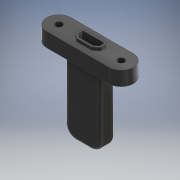
# Autodesk Inventor part: hdmi-panel-mount
Saved by Autodesk Inventor 2017 (Build 210142000, 142)
## iProperties
Created: 2020-10-05
Part Number: hdmi-panel-mount
Material: Generic
Document SubType Name: Modeling
Designer: Joe Ferner
Density: 1 g/cm^3
Appearance: Default
Author: Joe Ferner
Autodesk Inventor part; units mm, degrees
ref_plane "YZ Plane" through (0, 0, 0) normal (1, 0, 0) x (0, 1, 0)
ref_plane "XZ Plane" through (0, 0, 0) normal (0, 1, 0) x (-1, 0, 0)
ref_plane "XY Plane" through (0, 0, 0) normal (0, 0, 1) x (1, 0, 0)
sketch "Sketch1" plane through (0, 0, 0) normal (0, 0, 1) x (1, 0, 0)
  line L0 (0, 0) -> (43.8634, 0)
  line L1 (43.8634, 17.0268) -> (0, 17.0268)
  arc A0 (0, 17.0268) -> (0, 0) centre (0, 8.5134) ccw
  arc A1 (43.8634, 0) -> (43.8634, 17.0268) centre (43.8634, 8.5134) ccw
  circle A2 centre (0, 8.5134) radius 2.3193
  circle A3 centre (43.8634, 8.5134) radius 2.3193
  dimension "d0" = 43.8634
  dimension "d1" = 17.0268
  dimension "d2" = 4.6385
  constraints: 4 centre point, 4 end point, 4 point on circle, 4 tangent, 2 coincident, 1 equal radius, 1 horizontal, 1 parallel
  measures "d0" distance of L0.start L0.end
  measures "d1" distance between parallel lines of L1 L0
  measures "d2" diameter of A2
extrude "Extrusion1" add sketch "Sketch1" against normal blind 10
sketch "Sketch2" plane through (0, 0, 0) normal (0, 0, 1) x (1, 0, 0)
  line L0 (0, 0) -> (43.8634, 0) projected
  arc A0 (0, 17.0268) -> (0, 0) centre (0, 8.5134) ccw projected
  line L1 (15.7272, 6.9359) -> (16.5422, 6.0099)
  line L2 (17.1427, 5.7384) -> (26.7207, 5.7384)
  line L3 (27.3213, 6.0099) -> (28.1362, 6.9359)
  line L4 (28.3874, 7.0982) -> (28.867, 7.2458)
  line L5 (29.4317, 8.0104) -> (29.4317, 10.4884)
  line L6 (28.6317, 11.2884) -> (15.2317, 11.2884)
  line L7 (14.4317, 10.4884) -> (14.4317, 8.0104)
  line L8 (14.9965, 7.2458) -> (15.476, 7.0982)
  line L9 (43.8634, 17.0268) -> (0, 17.0268) projected
  arc A1 (15.2317, 11.2884) -> (14.4317, 10.4884) centre (15.2317, 10.4884) ccw
  arc A2 (29.4317, 10.4884) -> (28.6317, 11.2884) centre (28.6317, 10.4884) ccw
  arc A3 (14.4317, 8.0104) -> (14.9965, 7.2458) centre (15.2317, 8.0104) ccw
  arc A4 (28.867, 7.2458) -> (29.4317, 8.0104) centre (28.6317, 8.0104) ccw
  arc A5 (15.7272, 6.9359) -> (15.476, 7.0982) centre (15.3143, 6.5725) ccw
  arc A6 (28.3874, 7.0982) -> (28.1362, 6.9359) centre (28.5491, 6.5725) ccw
  arc A7 (16.5422, 6.0099) -> (17.1427, 5.7384) centre (17.1427, 6.5384) ccw
  arc A8 (26.7207, 5.7384) -> (27.3213, 6.0099) centre (26.7207, 6.5384) ccw
  line L10 (15.2317, 12.6529) -> (28.6317, 12.6529)
  arc A9 (30.7962, 10.4884) -> (28.6317, 12.6529) centre (28.6317, 10.4884) ccw
  line L11 (30.7962, 10.4884) -> (30.7962, 8.0104)
  arc A10 (29.2682, 5.9416) -> (30.7962, 8.0104) centre (28.6317, 8.0104) ccw
  line L12 (29.2682, 5.9416) -> (29.0086, 5.8617)
  line L13 (29.0086, 5.8617) -> (28.3456, 5.1084)
  arc A11 (26.7207, 4.3739) -> (28.3456, 5.1084) centre (26.7207, 6.5384) ccw
  line L14 (26.7207, 4.3739) -> (17.1427, 4.3739)
  arc A12 (15.5178, 5.1084) -> (17.1427, 4.3739) centre (17.1427, 6.5384) ccw
  line L15 (15.5178, 5.1084) -> (14.8549, 5.8617)
  line L16 (14.8549, 5.8617) -> (14.5953, 5.9416)
  arc A13 (13.0672, 8.0104) -> (14.5953, 5.9416) centre (15.2317, 8.0104) ccw
  line L17 (13.0672, 8.0104) -> (13.0672, 10.4884)
  arc A14 (15.2317, 12.6529) -> (13.0672, 10.4884) centre (15.2317, 10.4884) ccw
  point P0 (15.6245, 7.0525)
  point P1 (16.7811, 5.7384)
  point P2 (27.0824, 5.7384)
  point P3 (28.2389, 7.0525)
  point P4 (29.4317, 7.4195)
  point P5 (29.4317, 11.2884)
  point P6 (14.4317, 11.2884)
  point P7 (14.4317, 7.4195)
  dimension "d25" = 15
  dimension "d26" = 5.55
  dimension "d27" = 14.4317
  dimension "d28" = 5.7384
  dimension "d29" = 0.8
  dimension "d30" = 0.8
  dimension "d32" = 107.1
  dimension "d34" = 107.1
  dimension "d35" = 41.35
  dimension "d36" = 41.35
  dimension "d37" = 0.55
  dimension "d38" = 0.8
  dimension "d39" = 2.711
  dimension "d40" = 2.711
  dimension "d42" = 2.478
  dimension "d43" = 2.478
  dimension "d44" = 1.3645
  constraints: 32 end point, 28 point on circle, 16 point on line, 16 tangent, 14 centre point, 4 equal radius, 4 parallel, 2 perpendicular, 13 other
  measures "d25" distance between parallel lines of L5 L7
  measures "d26" distance between parallel lines of L6 L2
  measures "d27" distance from line of A0.centre L7
  measures "d28" distance between parallel lines of L9 L6
  measures "d29" radius of A1
  measures "d30" radius of A3
  measures "d32" angle of L8 L7
  measures "d34" angle of L4 L5
  measures "d35" angle of L1 L7
  measures "d36" angle of L5 L3
  measures "d37" radius of A5
  measures "d38" radius of A7
  measures "d39" distance from line of L2.start L7
  measures "d40" distance from line of L2.end L5
  measures "d42" distance of L7.start L7.end
  measures "d43" distance of L5.start L5.end
  measures "d44" distance between parallel lines of L2 L14
extrude "Extrusion4" add sketch "Sketch2" along normal blind 2 contours A5 L8 A3 L7 A1 L6 A2 L5 A4 L4 A6 L3 A8 L2 A7 L1 | L10 A9 L11 A10 L12 L13 A11 L14 A12 L15 L16 A13 L17 A14
extrude "Extrusion5" cut sketch "Sketch2" against normal blind 4 and the other way blind 2 contours A5 L8 A3 L7 A1 L6 A2 L5 A4 L4 A6 L3 A8 L2 A7 L1
sketch "Sketch3" plane through (0, 0, -10) normal (0, 0, -1) x (-1, 0, 0)
  line L0 (-34.3974, 3.5063) -> (-9.466, 3.5063)
  line L1 (-9.466, 3.5063) -> (-9.466, 13.5205)
  line L2 (-9.466, 13.5205) -> (-34.3974, 13.5205)
  line L3 (-34.3974, 13.5205) -> (-34.3974, 3.5063)
  line L4 (0, 17.0268) -> (-43.8634, 17.0268) projected
  arc A0 (-43.8634, 17.0268) -> (-43.8634, 0) centre (-43.8634, 8.5134) ccw projected
  point P0 (0, 0)
  dimension "d47" = 24.9314
  dimension "d48" = 10.0143
  dimension "d49" = 3.5063
  dimension "d51" = 9.466
  constraints: 8 end point, 2 parallel, 1 horizontal, 1 perpendicular
  measures "d47" distance of L0.start L0.end
  measures "d48" distance of L2.end L0.start
  measures "d49" distance between parallel lines of L4 L2
  measures "d51" distance from line of A0.centre L3
extrude "Extrusion6" add sketch "Sketch3" along normal blind 50
sketch "Sketch4" plane through (9.466, 13.5205, -10) normal (0, 1, 0) x (1, 0, 0)
  line L0 (24.9314, 0) -> (24.9314, 50) projected
  line L1 (24.9314, 50) -> (0, 50) projected
  arc A0 (24.9314, 42.7781) -> (17.7094, 50) centre (17.7094, 42.7781) ccw
  arc A1 (7.2219, 50) -> (0, 42.7781) centre (7.2219, 42.7781) ccw
  line L2 (24.9314, 42.7781) -> (24.9314, 50)
  line L3 (24.9314, 50) -> (17.7094, 50)
  line L4 (7.2219, 50) -> (0, 50)
  line L5 (0, 50) -> (0, 42.7781)
  line L6 (0, 0) -> (0, 50) projected
  point P0 (-9.466, -10)
  dimension "d54" = 7.2219
  dimension "d55" = 7.2219
  dimension "d56" = 7.2219
  dimension "d57" = 7.2219
  dimension "d58" = 7.2219
  dimension "d59" = 7.2219
  constraints: 8 end point, 4 collinear, 4 point on circle, 3 point on line, 2 centre point, 1 vertical alignment
  measures "d54" distance of L0.end L3.end
  measures "d55" distance of L1.end L4.start
  measures "d56" distance of L1.end L5.end
  measures "d57" distance of L0.end L2.start
  measures "d58" radius of A0
  measures "d59" radius of A1
extrude "Extrusion7" cut sketch "Sketch4" against normal through all
fillet "Fillet1" radius 2 10 edges at (32.2821, 13.5205, -57.8847) (21.9317, 13.5205, -60) (11.5813, 13.5205, -57.8847) (9.466, 13.5205, -31.389) (34.3974, 13.5205, -31.389) (32.2821, 3.5063, -57.8847) (21.9317, 3.5063, -60) (11.5813, 3.5063, -57.8847) (9.466, 3.5063, -31.389) (34.3974, 3.5063, -31.389)
equation "\"d27\" = -0.5 * d25 + 0.5 * d0"
equation "\"d28\" = -0.5 * d26 + 0.5 * d1"
equation "\"d34\" = d32"
equation "\"d36\" = d35"
equation "\"d40\" = d39"
equation "\"d43\" = d42"
equation "\"d49\" = -0.5 * d48 + 0.5 * d1"
equation "\"d51\" = -0.5 * d47 + 0.5 * d0"
equation "\"d55\" = d54"
equation "\"d56\" = d54"
equation "\"d57\" = d54"
equation "\"d58\" = d54"
equation "\"d59\" = d54"
body "Solid1"
